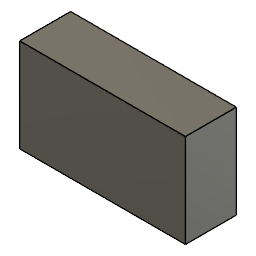
fuse+box+mock (Autodesk Fusion 360 design; units mm, degrees)
part number: 2026-02-08-15-27-38-561
Autodesk Fusion 360 part; units mm, degrees
sketch "Sketch1" plane through (0, 0, 0) normal (0, 0, 1) x (1, 0, 0)
  line L0 (-28.0698, 29.323) -> (95.7552, 29.323)
  line L1 (95.7552, 29.323) -> (95.7552, -40.527)
  line L2 (95.7552, -40.527) -> (-28.0698, -40.527)
  line L3 (-28.0698, -40.527) -> (-28.0698, 29.323)
  dimension "d1" = 123.825
  dimension "d2" = 69.85
  constraint horizontal L0
  constraint vertical L1
  constraint horizontal L2
  constraint vertical L3
  measures "d1" distance of L0.start L0.end
  measures "d2" distance of L0.start L2.end
extrude "Extrude1" add sketch "Sketch1" along normal blind 38.1
